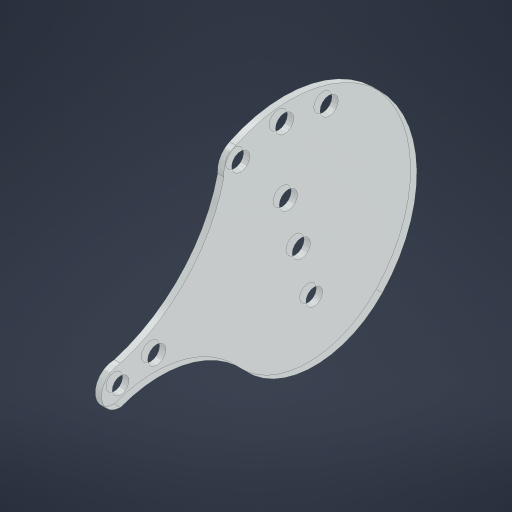
# Autodesk Inventor part: Odom Pod Poly
Saved by Autodesk Inventor 2023 (Build 270158000, 158)
## iProperties
Created: 2022-12-10
Part Number: Odom Pod Poly
Material: Polycarbonate, Clear
Document SubType Name: Modeling
Designer: nguye
Density: 1.2 g/cm^3
Appearance: Clear
Author: nguye
Autodesk Inventor part; units mm, degrees
ref_plane "YZ Plane" through (0, 0, 0) normal (1, 0, 0) x (0, 1, 0)
ref_plane "XZ Plane" through (0, 0, 0) normal (0, 1, 0) x (-1, 0, 0)
ref_plane "XY Plane" through (0, 0, 0) normal (0, 0, 1) x (1, 0, 0)
sketch "Sketch4" plane through (0, 0, 0) normal (1, 0, 0) x (0, 1, 0)
  line L0 (-0.177, -66.4213) -> (-12.877, -66.4213)
  line L1 (0, -49.1236) -> (-5.08, -49.1236)
  circle A0 centre (-5.08, -49.1236) radius 2.1209
  line L2 (-5.08, -49.1236) -> (7.1876, -45.838)
  arc A1 (-12.7, -31.6611) -> (-12.877, -66.4213) centre (3.3882, -49.1236) ccw
  circle A2 centre (7.1876, -45.838) radius 2.3114
  arc A3 (-12.877, -66.4213) -> (38.1002, -29.2262) centre (9.1157, -43.0325) ccw
  circle A4 centre (19.4552, -42.5523) radius 2.3114
  line L3 (7.1876, -45.838) -> (19.4552, -42.5523)
  line L4 (38.1695, -29.2174) -> (33.9062, -30.4753)
  circle A5 centre (34.972, -52.8945) radius 2.3114
  circle A6 centre (36.7356, -41.6045) radius 2.3114
  arc A7 (39.2694, -49.6585) -> (39.5231, -48.5235) centre (33.2252, -47.7117) ccw
  line L5 (39.2474, -54.1108) -> (34.972, -52.8945)
  line L6 (41.1789, -41.481) -> (36.7356, -41.6045)
  circle A8 centre (33.9062, -30.4753) radius 2.3114
  arc A9 (38.1002, -29.2262) -> (32.6481, -26.212) centre (33.2894, -31.4901) ccw
  line L7 (33.9062, -30.4753) -> (32.6481, -26.212)
  arc A10 (-12.7, -31.6611) -> (-4.8514, 0) centre (-31.4487, -10.21) ccw
  line L8 (2.3114, 0) -> (4.8514, 0)
  arc A11 (4.8514, 0) -> (0, 4.8514) centre (0, 0) ccw
  arc A12 (0, 4.8514) -> (-4.8514, 0) centre (0, 0) ccw
  arc A13 (4.8514, 0) -> (32.6481, -26.212) centre (41.1134, 10.6096) ccw
  circle A14 centre (0, 0) radius 2.1209
  circle A15 centre (2.1209, -9.1751) radius 2.3114
  point P0 (38.105, -29.2364)
  point P1 (36.1231, -29.8211)
  point P2 (33.2519, -28.2584)
  dimension "d110" = 2.54
  dimension "d111" = 4.8514
  dimension "d112" = 5.08
  dimension "d113" = 12.7
  dimension "d114" = 6.35
  dimension "d115" = 4.445
  dimension "d116" = 4.6228
  dimension "d117" = 4.2418
  dimension "d118" = 4.445
  dimension "d119" = 12.7
  dimension "d120" = 12.7
  dimension "d121" = 4.6228
  dimension "d122" = 4.6228
  dimension "d123" = 4.445
  dimension "d124" = 4.6228
  dimension "d125" = 4.445
  dimension "d126" = 4.6228
  dimension "d127" = 4.2418
  dimension "d128" = 4.6228
  constraints: 18 end point, 17 point on circle, 16 centre point, 9 coincident, 2 horizontal, 1 point on line, 1 tangent
  measures "d110" distance of L8.start L8.end
  measures "d111" radius of A12
  measures "d112" distance of L1.start L1.end
  measures "d113" distance of L0.start L0.end
  measures "d114" radius of A7
  measures "d115" distance of L4.start L4.end
  measures "d116" diameter of A8
  measures "d117" diameter of A0
  measures "d118" distance of L7.start L7.end
  measures "d119" distance of L2.start L2.end
  measures "d120" distance of L2.end L3.end
  measures "d121" diameter of A2
  measures "d122" diameter of A4
  measures "d123" distance of L5.start L5.end
  measures "d124" diameter of A5
  measures "d125" distance of L6.start L6.end
  measures "d126" diameter of A6
  measures "d127" diameter of A14
  measures "d128" diameter of A15
extrude "Extrusion4" add sketch "Sketch4" along normal blind 1.5875 contours A10 A12 A11 A13 L7 A8 L4 A3 A1 | L4 A8 L7 A9 A3
body "Solid1"
